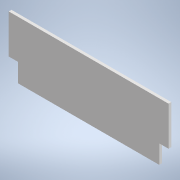
# Autodesk Inventor part: Array de sensores
Saved by Autodesk Inventor 2020 (Build 240168000, 168)
## iProperties
Created: 2020-04-22
Part Number: Array de sensores
Material: Genérico
Document SubType Name: Modeling
Designer: gi-se
Density: 1 g/cm^3
Appearance: Padrão
Author: gi-se
Autodesk Inventor part; units mm, degrees
ref_plane "YZ Plane" through (0, 0, 0) normal (1, 0, 0) x (0, 1, 0)
ref_plane "XZ Plane" through (0, 0, 0) normal (0, 1, 0) x (-1, 0, 0)
ref_plane "XY Plane" through (0, 0, 0) normal (0, 0, 1) x (1, 0, 0)
sketch "Esboço1" plane through (0, 0, 0) normal (0, 0, 1) x (1, 0, 0)
  line L0 (0, 0) -> (86, 0)
  line L1 (86, 0) -> (86, -21)
  line L2 (81, -31) -> (5, -31)
  line L3 (0, -21) -> (0, 0)
  line L4 (81, -31) -> (81, -21)
  line L5 (81, -21) -> (86, -21)
  line L6 (3, -21) -> (0, -21)
  line L7 (0, -21) -> (5, -21)
  line L8 (5, -21) -> (5, -31)
  constraints: 18 end point, 1 horizontal, 1 perpendicular, 1 point on line
extrude "Extrusão1" add sketch "Esboço1" along normal blind 1.5
